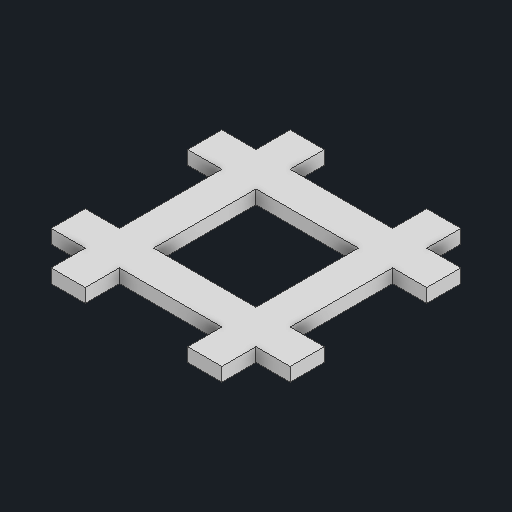
# Autodesk Inventor part: 110033226_ipt_27_騎樓梁架頂
Saved by Autodesk Inventor 2022 (Build 260153000, 153)
## iProperties
Created: 2022-06-24
Part Number: 110033226_ipt_27_騎樓梁架頂
Material: 一般
Document SubType Name: Modeling
Designer: User
Density: 1 g/cm^3
Appearance: 預設
Author: User
Autodesk Inventor part; units mm, degrees
ref_plane "YZ Plane" through (0, 0, 0) normal (1, 0, 0) x (0, 1, 0)
ref_plane "XZ Plane" through (0, 0, 0) normal (0, 1, 0) x (-1, 0, 0)
ref_plane "XY Plane" through (0, 0, 0) normal (0, 0, 1) x (1, 0, 0)
sketch "草圖1" plane through (0, 0, 0) normal (0, 1, 0) x (-1, 0, 0)
  line L0 (12.5, 12.5) -> (-12.5, 12.5) construction
  line L1 (-12.5, 12.5) -> (-12.5, -12.5) construction
  line L2 (-12.5, -12.5) -> (12.5, -12.5) construction
  line L3 (12.5, -12.5) -> (12.5, 12.5) construction
  circle A0 centre (10, 10) radius 1.7
  circle A1 centre (-10, 10) radius 1.7
  circle A2 centre (-10, -10) radius 1.7
  circle A3 centre (10, -10) radius 1.7
  line L4 (12.5, 12.5) -> (12.5, 17.5)
  line L5 (12.5, 17.5) -> (7.5, 17.5)
  line L6 (7.5, 17.5) -> (7.5, 12.5)
  line L7 (7.5, 12.5) -> (-7.5, 12.5)
  line L8 (12.5, 12.5) -> (17.5, 12.5)
  line L9 (17.5, 12.5) -> (17.5, 7.5)
  line L10 (17.5, 7.5) -> (12.5, 7.5)
  line L11 (12.5, 7.5) -> (12.5, 0)
  line L12 (-7.5, 12.5) -> (0, 12.5)
  line L13 (-7.5, 17.5) -> (-7.5, 12.5)
  line L14 (-12.5, 17.5) -> (-7.5, 17.5)
  line L15 (-12.5, 12.5) -> (-12.5, 17.5)
  line L16 (-12.5, 12.5) -> (-17.5, 12.5)
  line L17 (-17.5, 12.5) -> (-17.5, 7.5)
  line L18 (-17.5, 7.5) -> (-12.5, 7.5)
  line L19 (-12.5, 7.5) -> (-12.5, -7.5)
  line L20 (-12.5, -7.5) -> (-12.5, 0)
  line L21 (-17.5, -7.5) -> (-12.5, -7.5)
  line L22 (-17.5, -12.5) -> (-17.5, -7.5)
  line L23 (-12.5, -12.5) -> (-17.5, -12.5)
  line L24 (-12.5, -12.5) -> (-12.5, -17.5)
  line L25 (-12.5, -17.5) -> (-7.5, -17.5)
  line L26 (-7.5, -17.5) -> (-7.5, -12.5)
  line L27 (-7.5, -12.5) -> (7.5, -12.5)
  line L28 (7.5, -12.5) -> (0, -12.5)
  line L29 (7.5, -17.5) -> (7.5, -12.5)
  line L30 (12.5, -17.5) -> (7.5, -17.5)
  line L31 (12.5, -12.5) -> (12.5, -17.5)
  line L32 (12.5, -12.5) -> (17.5, -12.5)
  line L33 (17.5, -12.5) -> (17.5, -7.5)
  line L34 (17.5, -7.5) -> (12.5, -7.5)
  line L35 (12.5, -7.5) -> (12.5, 7.5)
  line L36 (7.5, 7.5) -> (-7.5, 7.5)
  line L37 (-7.5, 7.5) -> (-7.5, -7.5)
  line L38 (-7.5, -7.5) -> (7.5, -7.5)
  line L39 (7.5, -7.5) -> (7.5, 7.5)
  point P0 (0, 0)
  point P1 (0, -12.5)
  point P2 (7.5, 0)
  point P3 (0, -7.5)
  point P4 (12.5, 0)
  dimension "d0" = 25
  dimension "d1" = 25
  dimension "d2" = 3.4
  dimension "d3" = 2.5
  dimension "d4" = 2.5
  dimension "d7" = 360
  dimension "d9" = 5
  dimension "d10" = 5
  dimension "d11" = 5
  dimension "d12" = 15
  dimension "d13" = 5
  dimension "d14" = 5
  dimension "d15" = 5
  dimension "d18" = 360
  dimension "d20" = 15
  dimension "d21" = 15
  constraints: 80 end point, 4 centre point, 4 midpoint, 4 parallel, 4 perpendicular, 3 horizontal, 3 point on line, 2 horizontal alignment, 2 vertical alignment, 1 vertical, 78 other
  measures "d0" distance of L2.end L1.end
  measures "d1" distance of L1.end L0.end
  measures "d2" diameter of A0
  measures "d3" distance from line of L3 A0.centre
  measures "d4" distance from line of L0 A0.centre
  measures "d9" distance of L0.start L4.end
  measures "d10" distance of L4.end L5.end
  measures "d11" distance of L5.end L6.end
  measures "d12" distance of L6.end L7.end
  measures "d13" distance of L0.start L8.end
  measures "d14" distance of L8.end L9.end
  measures "d15" distance of L9.end L10.end
  measures "d20" distance of L38.end L37.end
  measures "d21" distance of L37.end L36.end
extrude "擠出1" add sketch "草圖1" along normal blind 2 contours A0 | A1 | A2 | A3 | L8 L9 L10 L11 L35 L34 L33 L32 L31 L30 L29 L27 L26 L25 L24 L23 L22 L21 L19 L18 L17 L16 L15 L14 L13 L7 L6 L5 L4
extrude "擠出2" cut sketch "草圖1" along normal blind 1.5 contours A0 | A1 | A2 | A3
